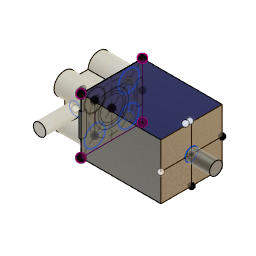
_ 5V mini valve v1 (Autodesk Fusion 360 design; units mm, degrees)
Autodesk Fusion 360 part; units mm, degrees
sketch "Sketch1" plane through (0, 0, 0) normal (1, 0, 0) x (0, 0, -1)
  line L0 (0, 0) -> (-12.9, 0)
  line L1 (-12.9, 0) -> (-12.9, 14.3)
  line L2 (-12.9, 14.3) -> (0, 14.3)
  line L3 (0, 14.3) -> (0, 0)
  dimension "d86" = 12.9
  dimension "d87" = 14.3
  constraint horizontal L0
  constraint vertical L1
  constraint horizontal L2
  constraint vertical L3
  constraint coincident L0.start L3.end
  measures "d86" distance of L0.start L0.end
  measures "d87" distance of L0.start L2.end
extrude "Extrude1" add sketch "Sketch1" along normal blind 18.6 makes body 1
sketch "end with metal pin" plane through (18.6, 0, 0) normal (1, 0, 0) x (0, 0, -1)
  line L0 (0, 14.3) -> (-12.9, 14.3)
  line L1 (-12.9, 14.3) -> (-12.9, 0)
  line L2 (-12.9, 0) -> (0, 0)
  line L3 (0, 0) -> (0, 14.3)
  line L4 (-6.45, 14.3) -> (-6.45, 0)
  line L5 (0, 7.15) -> (-12.9, 7.15)
  circle A0 centre (-6.45, 7.15) radius 1.5
  point P0 (-6.45, 14.3)
  point P1 (0, 7.15)
  dimension "d91" = 3
  constraint midpoint L0 P0
  constraint midpoint L3 P1
  constraint coincident P0 L4.start
  constraint perpendicular L0 L4
  constraint coincident P1 L5.start
  constraint midpoint L1 L5.end
  constraint midpoint L4 A0.centre
  measures "d91" diameter of A0
extrude "Extrude2" add sketch "end with metal pin" along normal blind 5.7 contours L4 L5 A0 | L4 L5 A0 | L4 L5 A0 | L4 L5 A0 bodies 1
sketch "base for plastic mountplate with screw holes" plane through (0, 0, 0) normal (-1, 0, 0) x (0, 0, 1)
  line L0 (12.9, 14.3) -> (0, 14.3)
  line L1 (0, 14.3) -> (0, 0)
  line L2 (0, 0) -> (12.9, 0)
  line L3 (12.9, 0) -> (12.9, 14.3)
  circle A0 centre (2.8664, 11.1225) radius 2.5
  line L4 (0, 0) -> (0, 14.3)
  line L5 (0, 14.3) -> (12.9, 14.3)
  circle A1 centre (10.0336, 11.1225) radius 2.5
  line L6 (12.9, 0) -> (12.9, 14.3)
  circle A2 centre (10.0336, 3.1775) radius 2.5
  circle A3 centre (2.8584, 3.1775) radius 2.5
  line L7 (0, 0) -> (12.9, 0)
  line L8 (12.9, 14.3) -> (0, 14.3)
  line L9 (0, 14.3) -> (0, 0)
  line L10 (10.0336, 11.1225) -> (2.8584, 11.1225)
  line L11 (2.8584, 11.1225) -> (2.8584, 3.1775)
  line L12 (2.8584, 3.1775) -> (10.0336, 3.1775)
  line L13 (10.0336, 3.1775) -> (10.0336, 11.1225)
  circle A4 centre (10.0336, 11.1225) radius 2.3
  circle A5 centre (2.8664, 11.1225) radius 2.3
  circle A6 centre (2.8584, 3.1775) radius 2.3
  circle A7 centre (10.0336, 3.1775) radius 2.3
  line L14 (12.9, 0) -> (0, 14.3) construction
  line L15 (12.9, 14.3) -> (0, 0) construction
  circle A8 centre (6.45, 7.15) radius 3.9
  circle A9 centre (6.45, 7.15) radius 3.15
  circle A10 centre (6.45, 7.15) radius 2.65
  circle A11 centre (2.8664, 11.1225) radius 0.925
  circle A12 centre (10.0336, 3.1775) radius 0.925
  circle A13 centre (6.45, 7.15) radius 5.35 construction
  point P0 (6.45, 7.15)
  point P1 (10.0336, 11.1225)
  point P2 (2.8664, 11.1225)
  point P3 (2.8664, 3.1775)
  point P4 (10.0336, 3.1775)
  dimension "d94" = 5
  dimension "d95" = 5
  dimension "d96" = 5
  dimension "d97" = 5
  dimension "d98" = 0.2
  dimension "d101" = 0.2
  dimension "d133" = 7.8
  dimension "d134" = 0.75
  dimension "d135" = 1.25
  dimension "d140" = 1.85
  dimension "d141" = 1.85
  dimension "d249" = 10.7
  dimension "d250" = 0.2
  constraint horizontal L10
  constraint vertical L11
  constraint horizontal L12
  constraint vertical L13
  constraint coincident A3.centre L11.end
  constraint coincident P1 A1.centre
  constraint coincident L2.end L3.start
  constraint coincident L0.end L1.start
  constraint coincident L0.start L3.end
  constraint coincident L1.end L2.start
  constraint midpoint L15 P0
  constraint coincident P0 A8.centre
  constraint coincident P2 A13
  constraint concentric A5 A11
  constraint concentric A0 A5
  constraint concentric A3 A6
  constraint concentric A7 A12
  constraint concentric A10 A13
  constraint coincident A13 P1
  constraint coincident L15 P1
  constraint coincident A13 P2
  constraint coincident L14 P2
  constraint coincident A13 P3
  constraint coincident L15 P3
  constraint coincident A13 P4
  constraint coincident L14 P4
  constraint coincident P4 A2.centre
  constraint coincident P2 L10
  measures "d94" diameter of A0
  measures "d95" diameter of A1
  measures "d96" diameter of A3
  measures "d97" diameter of A2
  measures "d133" diameter of A8
  measures "d140" diameter of A11
  measures "d141" diameter of A12
  measures "d249" diameter of A13
  measures "d250" distance of A0 A5
extrude "Extrude10" add sketch "base for plastic mountplate with screw holes" along normal blind 0.5 separate body contours A0 A3 L11 A8 | A0 A1 A8 A9 | A0 A5 A8 A9 | A0 L11 A5 A8 A9 | A0 A3 L11 A9 | A1 A4 A8 A9 | A5 A8 A9 | A3 L11 A6 A8 A9 | A4 A8 A9 | A1 A2 L13 A8 | A3 A6 A8 A9 | A2 A3 A8 A9 | A6 A8 A9 | A1 L13 A4 A8 A9 | A1 A2 L13 A9 | A2 A7 A8 A9 | A2 L13 A7 A8 A9 | A7 A8 A9 makes body 2
extrude "Extrude11" add sketch "base for plastic mountplate with screw holes" along normal blind 2.55 separate body contours A0 A1 A2 A3 A9 | A0 A5 A9 | A1 A4 A9 | A5 A9 | A3 A6 A9 | A4 A9 | A6 A9 | A2 A7 A9 | A7 A9 makes body 3
extrude "Extrude12" cut sketch "base for plastic mountplate with screw holes" against normal blind 2 contours L10 L11 A11 | L10 L11 A11 | L12 L13 A12 | L12 L13 A12 bodies 1
sketch "Sketch3" plane through (0, 0, 0) normal (1, 0, 0) x (0, 0, -1)
  line L0 (-3.675, 14.3) -> (-9.225, 14.3)
  line L1 (-9.225, 14.3) -> (-9.225, 13.05)
  line L2 (-9.225, 13.05) -> (-3.675, 13.05)
  line L3 (-3.675, 13.05) -> (-3.675, 14.3)
  line L4 (-12.9, 14.3) -> (0, 14.3)
  line L5 (0, 14.3) -> (0, 0)
  line L6 (-12.9, 0) -> (-12.9, 14.3)
  line L7 (0, 7.15) -> (-12.9, 7.15) construction
  line L8 (-9.225, 1.25) -> (-3.675, 1.25)
  line L9 (-3.675, 1.25) -> (-3.675, 0)
  line L10 (-3.675, 0) -> (-9.225, 0)
  line L11 (-9.225, 0) -> (-9.225, 1.25)
  point P0 (-6.45, 14.3)
  dimension "d278" = 1.25
  dimension "d279" = 5.55
  constraint horizontal L0
  constraint vertical L1
  constraint horizontal L2
  constraint vertical L3
  constraint midpoint L0 P0
  constraint midpoint P0 L4
  constraint midpoint L5 L7.start
  constraint midpoint L6 L7.end
  constraint symmetric L0.start L7 L9.end
  constraint symmetric L0.end L7 L10.end
  constraint symmetric L1.end L7 L8.start
  constraint symmetric L2.end L7 L8.end
  measures "d278" distance of L0 L2
  measures "d279" distance of L1 L3
extrude "Extrude14" add sketch "Sketch3" against normal blind 0.5 bodies 1
extrude "Extrude3" add sketch "base for plastic mountplate with screw holes" along normal blind 7 separate body contours A0 L10 L11 A5 A8 | A0 A1 L10 A8 | A0 L10 A5 A8 | A0 L11 A8 | A0 A1 A8 A9 | A0 A5 A8 A9 | A1 L10 A4 A8 | A1 L10 L13 A4 A8 | A0 L11 A5 A8 A9 | A0 A3 L11 A9 | L11 A5 A8 | A3 L11 L12 A6 A8 | A3 L11 A8 | A0 A1 A2 A3 A9 | A0 A5 A9 | A1 A4 A8 A9 | A3 L11 A6 A8 A9 | A3 L12 A6 A8 | A2 A3 L12 A8 | L11 A6 A8 | A1 A4 A9 | A1 L13 A8 | A3 A6 A9 | A3 A6 A8 A9 | A2 A3 A8 A9 | A2 L12 L13 A7 A8 | A2 L12 A7 A8 | A1 L13 A4 A8 A9 | A1 A2 L13 A9 | L13 A4 A8 | A2 A7 A8 A9 | A2 L13 A7 A8 A9 | A2 L13 A8 | A2 A7 A9 | L13 A7 A8 | A10 makes body 4
sketch "Sketch10" plane through (-7, 0, 0) normal (-1, 0, 0) x (0, 0, 1)
  circle A0 centre (10.0336, 3.1775) radius 2.3
  circle A1 centre (2.8584, 3.1775) radius 2.3
  circle A2 centre (10.0336, 11.1225) radius 2.3
  circle A3 centre (2.8664, 11.1225) radius 2.3
  arc A4 (7.5336, 3.1775) -> (10.0336, 5.6775) centre (10.0336, 3.1775) ccw
  line L0 (10.0336, 5.6775) -> (10.0336, 8.6225)
  arc A5 (10.0336, 8.6225) -> (7.5336, 11.1225) centre (10.0336, 11.1225) ccw
  line L1 (7.5336, 11.1225) -> (5.3664, 11.1225)
  arc A6 (5.3664, 11.1225) -> (2.8584, 8.6225) centre (2.8664, 11.1225) ccw
  line L2 (2.8584, 8.6225) -> (2.8584, 5.6775)
  arc A7 (2.8584, 5.6775) -> (5.3584, 3.1775) centre (2.8584, 3.1775) ccw
  line L3 (5.3584, 3.1775) -> (7.5336, 3.1775)
  circle A8 centre (6.45, 7.15) radius 0.95
  point P0 (6.45, 7.15)
  dimension "d126" = 1.9
  constraint coincident P0 A8.centre
  measures "d126" diameter of A8
extrude "Extrude9" add sketch "Sketch10" along normal blind 4.5 contours A8 bodies 4
sketch "Sketch4" plane through (0, 3.1775, 0) normal (0, -1, 0) x (1, 0, 0)
  line L0 (0, 7.5336) -> (-7, 7.5336)
  line L1 (-7, 7.5336) -> (-7, 5.3584)
  line L2 (-7, 5.3584) -> (0, 5.3584)
  circle A0 centre (-4.4635, 6.0836) radius 1.45
  line L3 (0, 5.3584) -> (0, 7.5336)
  constraint tangent L0 A0
extrude "Extrude4" add sketch "Sketch4" along normal blind 8.4 contours L2 A0 | L2 A0 bodies 4
sketch "Sketch7" plane through (18.6, 0, 0) normal (1, 0, 0) x (0, 0, -1)
  circle A0 centre (-6.45, 7.15) radius 1.5
  line L0 (0, 14.3) -> (-12.9, 14.3)
  line L1 (-12.9, 14.3) -> (-12.9, 0)
  line L2 (-12.9, 0) -> (0, 0)
  line L3 (0, 0) -> (0, 14.3)
  circle A1 centre (-13.3605, 5.7109) radius 0.5
  circle A2 centre (-13.3531, 6.7768) radius 0.5
  dimension "d106" = 1
  dimension "d107" = 1
  measures "d106" diameter of A1
  measures "d107" diameter of A2
named bodies: "coil house", "rubber gasket", "Inner plastic cylinder", "plastic air house"
